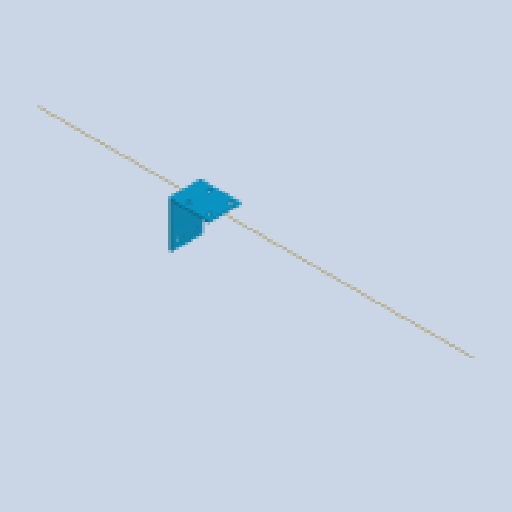
# Autodesk Inventor part: крепление энкодера
Saved by Autodesk Inventor 2024.2 (Build 282272000, 272)
## iProperties
Created: 2025-11-27
Part Number: крепление энкодера
Material: Типовые
Document SubType Name: Modeling
Designer: katya_notebook
Density: 1 g/cm^3
Appearance: Небесно-голубой
Author: katya_notebook
Autodesk Inventor part; units mm, degrees
ref_plane "YZ Plane" through (0, 0, 0) normal (1, 0, 0) x (0, 1, 0)
ref_plane "XZ Plane" through (0, 0, 0) normal (0, 1, 0) x (-1, 0, 0)
ref_plane "XY Plane" through (0, 0, 0) normal (0, 0, 1) x (1, 0, 0)
sketch "Эскиз1" plane through (0, 0, 0) normal (0, 1, 0) x (-1, 0, 0)
  line L0 (-15, -12) -> (15, -12)
  line L1 (15, -12) -> (15, 12)
  line L2 (15, 12) -> (-15, 12)
  line L3 (-15, 12) -> (-15, -12)
  line L4 (-15, -12) -> (15, 12) construction
  line L5 (15, -12) -> (-15, 12) construction
  point P0 (0, 0)
  dimension "d0" = 24
  dimension "d1" = 30
  constraints: 12 end point, 2 midpoint, 2 parallel, 1 horizontal, 1 perpendicular
  measures "d0" distance of L0.end L1.end
  measures "d1" distance of L1.end L2.end
extrude "Выдавливание1" add sketch "Эскиз1" along normal blind 2
sketch "Эскиз2" plane through (0, 2, 0) normal (0, 1, 0) x (1, 0, 0)
  circle A0 centre (11.5163, 7.8272) radius 2 projected
  circle A1 centre (11.5163, -7.8272) radius 2 projected
  circle A2 centre (-4.4163, -7.8272) radius 2 projected
  circle A3 centre (-4.4163, 7.8272) radius 2 projected
  point P0 (0, 0)
extrude "Выдавливание2" cut sketch "Эскиз2" against normal blind 2
sketch "Эскиз3" plane through (0, 0, 0) normal (0, -1, 0) x (1, 0, 0)
  line L0 (15, -12) -> (-15, -12) projected
  line L1 (-15, 12) -> (15, 12) projected
  line L2 (-15, -12) -> (-13, -12)
  line L3 (-13, -12) -> (-13, 12)
  line L4 (-13, 12) -> (-15, 12)
  line L5 (-15, 12) -> (-15, -12)
  point P0 (0, 0)
  dimension "d6" = 2
  constraints: 8 end point, 2 parallel, 1 horizontal, 1 perpendicular, 1 point on line
  measures "d6" distance of L1.start L3.end
ref_plane "РабПлоскость1" through (-96.45, -32.75, -191.5) normal (0, 1, 0) x (0, 0, 1)
extrude "Выдавливание3" add sketch "Эскиз3" along normal up to surface (32.75 mm away)
sketch "Эскиз4" plane through (-15, 2, -12) normal (-1, 0, 0) x (0, 0, 1)
  line L0 (15.35, -27.95) -> (20.15, -27.95)
  line L1 (20.15, -27.95) -> (20.15, -29.75)
  line L2 (20.15, -29.75) -> (15.35, -29.75)
  line L3 (15.35, -29.75) -> (15.35, -27.95)
  line L4 (15.35, -27.95) -> (20.15, -29.75) construction
  line L5 (20.15, -27.95) -> (15.35, -29.75) construction
  line L6 (3.85, -27.95) -> (8.65, -27.95)
  line L7 (8.65, -27.95) -> (8.65, -29.75)
  line L8 (3.85, -29.75) -> (3.85, -27.95)
  line L9 (3.85, -27.95) -> (8.65, -29.75) construction
  line L10 (8.65, -27.95) -> (3.85, -29.75) construction
  line L11 (8.65, -29.75) -> (3.85, -29.75)
  line L12 (24, -2) -> (24, -34.75) projected
  line L13 (24, -34.75) -> (-0.0211, -34.75)
  line L14 (0, 0) -> (0, -34.75) projected
  line L15 (24, -34.75) -> (24, 0) projected
  line L16 (0, 0) -> (24, 0) projected
  line L17 (0, 0) -> (0, -34.75) projected
  line L18 (24, -34.75) -> (0, -34.75) projected
  point P0 (12, -2)
  point P1 (17.75, -28.85)
  point P2 (6.25, -28.85)
  dimension "d9" = 4.8
  dimension "d10" = 1.8
  dimension "d13" = 4.8
  dimension "d14" = 1.8
  dimension "d15" = 5
  dimension "d16" = 5
  dimension "d17" = 3.85
  dimension "d18" = 3.85
  constraints: 26 end point, 4 midpoint, 4 parallel, 3 horizontal, 2 perpendicular
  measures "d9" distance of L1.end L3.start
  measures "d10" distance of L3.start L0.start
  measures "d13" distance of L7.end L8.start
  measures "d14" distance of L8.start L6.start
  measures "d15" distance between parallel lines of L2 L13
  measures "d16" distance between parallel lines of L11 L13
  measures "d17" distance between parallel lines of L1 L12
  measures "d18" distance between parallel lines of L14 L8
extrude "Выдавливание5" cut sketch "Эскиз4" against normal blind 10 contours L0 L1 L2 L3 | L6 L7 L11 L8
sketch "Эскиз5" plane through (-15, -32.75, -12) normal (0, -1, 0) x (1, 0, 0)
  circle A0 centre (1, 6.25) radius 1 projected
  circle A1 centre (0.6388, 17.75) radius 1.3612 projected
  circle A2 centre (1, 6.25) radius 1
  circle A3 centre (0.6388, 17.75) radius 1.3612
  point P0 (15, 12)
  constraints: 2 centre point, 2 coincident, 2 concentric
extrude "Выдавливание6" cut sketch "Эскиз5" against normal blind 10
